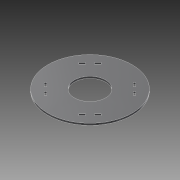
# Autodesk Inventor part: Диск_опорный_В5
Saved by Autodesk Inventor 2021.3 (Build 253353000, 353)
## iProperties
RuleStatus: InUse
Part Number: Диск_опорный_В5
Checked By: Якушев
Engr Approved By: Малов
Material: По умолчанию1
Document SubType Name: Modeling
Mfg Approved By: Судаков
Designer: Смирнов
Density: 1 g/cm^3
Appearance: Гладкий — нейтральный серый
AfterMaterialChange0: Материал
BeforeDocSave0: Материал
AfterAnyiPropertyChange0: Материал
Материал: По умолчанию1
Author: Смирнов
Autodesk Inventor part; units mm, degrees
ref_plane "YZ Plane" through (0, 0, 0) normal (1, 0, 0) x (0, 1, 0)
ref_plane "XZ Plane" through (0, 0, 0) normal (0, 1, 0) x (-1, 0, 0)
ref_plane "XY Plane" through (0, 0, 0) normal (0, 0, 1) x (1, 0, 0)
sketch "Эскиз1" plane through (0, 0, 0) normal (0, 0, 1) x (1, 0, 0)
  circle A0 centre (0, 0) radius 135
  dimension "d0" = 270
  constraints: 1 centre point, 1 coincident
  measures "d0" diameter of A0
extrude "Выдавливание1" add sketch "Эскиз1" along normal mid plane 6
sketch "Эскиз3" plane through (0, 0, -3) normal (0, 0, -1) x (-1, 0, 0)
  circle A0 centre (0, 0) radius 50
  dimension "d14" = 100
  constraints: 1 centre point, 1 coincident
  measures "d14" diameter of A0
extrude "Выдавливание2" cut sketch "Эскиз3" against normal through all
sketch "Эскиз4" plane through (0, 0, 3) normal (0, 0, 1) x (1, 0, 0)
  circle A0 centre (0, 0) radius 101 construction
  circle A1 centre (0, 101) radius 26.5 construction
  line L0 (0, 0) -> (118.5479, 118.5479) construction
  line L1 (0, 0) -> (0, 152.163) construction
  line L2 (86.9741, 51.6188) -> (51.6188, 86.9741)
  line L3 (51.6188, 86.9741) -> (55.8614, 91.2168)
  line L4 (55.8614, 91.2168) -> (91.2168, 55.8614)
  line L5 (91.2168, 55.8614) -> (86.9741, 51.6188)
  line L6 (86.9741, 51.6188) -> (55.8614, 91.2168) construction
  line L7 (51.6188, 86.9741) -> (91.2168, 55.8614) construction
  line L8 (66.468, 80.6102) -> (62.2254, 76.3675)
  line L9 (80.6102, 66.468) -> (76.3675, 62.2254)
  point P0 (71.4178, 71.4178)
  dimension "d17" = 202
  dimension "d18" = 53
  dimension "d19" = 45
  dimension "d20" = 6
  dimension "d21" = 50
  dimension "d22" = 15
  constraints: 20 end point, 5 point on line, 3 parallel, 2 centre point, 2 midpoint, 2 perpendicular, 2 point on circle, 1 coincident, 1 vertical, 1 vertical alignment, 1 other
  measures "d17" diameter of A0
  measures "d18" diameter of A1
  measures "d19" angle of L0 L1
  measures "d20" distance of L4.end L2.start
  measures "d21" distance of L3.end L4.end
  measures "d22" distance between parallel lines of L8 L3
extrude "Выдавливание3" cut sketch "Эскиз4" against normal through all contours L2 L9 L4 L5 | L2 L3 L4 L8
pattern_circular "Круговой массив2" count 4 over 360 about axis through (0, 0, 0) along (0, 0, 1) of "Выдавливание3"
